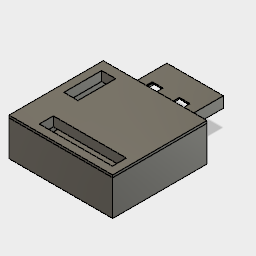
DigiCase (Autodesk Fusion 360 design; units mm, degrees)
Autodesk Fusion 360 part; units mm, degrees
sketch "Sketch1" plane through (0, 0, 0) normal (0, 1, 0) x (1, 0, 0)
  line L0 (0, 0) -> (-22, 0)
  line L1 (-22, 0) -> (-22, 20)
  line L2 (-22, 20) -> (-18, 20)
  line L3 (-18, 20) -> (-17, 20)
  line L4 (-5, 20) -> (0, 20)
  line L5 (0, 20) -> (0, 0)
  line L6 (-17, 20) -> (-5, 20)
  line L7 (-7.1, 21.5) -> (-7.1, 23.5)
  line L8 (-7.1, 23.5) -> (-9.35, 23.5)
  line L9 (-9.35, 23.5) -> (-9.35, 21.499)
  line L10 (-9.35, 21.499) -> (-7.1, 21.5)
  line L11 (-15.1, 21.5) -> (-15.1009, 23.4983)
  line L12 (-15.1009, 23.4983) -> (-12.8549, 23.4993)
  line L13 (-12.8549, 23.4993) -> (-12.854, 21.5032)
  line L14 (-12.854, 21.5032) -> (-15.1, 21.5)
  line L15 (-5.3006, 28.5) -> (-5.3006, 20)
  line L16 (-16.6958, 28.5) -> (-16.6958, 20)
  line L17 (-1.3, 19.5) -> (-1.3, 1.3)
  line L18 (-1.3, 1.3) -> (-20.7, 1.3)
  line L19 (-20.7, 1.3) -> (-20.7, 19.5)
  line L20 (-17.139, 1.5925) -> (-17.139, 4.5608)
  line L21 (-17.139, 4.5608) -> (-1.6625, 4.5608)
  line L22 (-1.6625, 4.5608) -> (-1.6625, 1.6)
  line L23 (-1.6625, 1.6) -> (-17.139, 1.5925)
  line L24 (-20.3439, 10.0007) -> (-20.3439, 18)
  line L25 (-20.3439, 18) -> (-17.3585, 18)
  line L26 (-17.3585, 18) -> (-17.3585, 10)
  line L27 (-17.3585, 10) -> (-20.3439, 10.0007)
  line L28 (-20.7, 19.5) -> (-1.3, 19.5)
  line L29 (-4.9026, 20) -> (-4.9026, 19.5)
  line L30 (-17.1025, 20) -> (-17.1025, 19.5)
  line L31 (-17, 20) -> (-17, 28.5)
  line L32 (-5, 20) -> (-5, 28.5)
  line L33 (-5, 28.5) -> (-17, 28.5)
  constraint perpendicular L0 L1
  constraint perpendicular L1 L2
  constraint perpendicular L1 L3
  constraint perpendicular L0 L5
  constraint coincident L6
  constraint perpendicular L6 L15
  constraint perpendicular L6 L16
  constraint perpendicular L17 L18
  constraint perpendicular L18 L19
  constraint vertical L20
  constraint perpendicular L20 L21
  constraint perpendicular L21 L22
  constraint perpendicular L24 L25
  constraint perpendicular L25 L26
  constraint coincident L4
  constraint coincident L3
  constraint coincident L28
  constraint perpendicular L28 L29
  constraint perpendicular L28 L30
  constraint perpendicular L6 L32
extrude "Extrude1" add sketch "Sketch1" along normal blind 0.5 contours L0 L1 L2 L3 L4 L5 L17 L18 L19 L28 L29 L30 | L3 L4 L6 L28 L29 L30 | L17 L18 L19 L28 makes body 1
extrude "Extrude2" add sketch "Sketch1" against normal blind 1.5 contours L17 L18 L19 L28 bodies 1
extrude "Extrude5" add sketch "Sketch1" along normal blind 1.5 separate body contours L0 L1 L2 L3 L4 L5 L17 L18 L19 L28 L29 L30 | L3 L4 L6 L28 L29 L30 | L17 L18 L19 L28 | L20 L21 L22 L23 | L24 L25 L26 L27 makes body 2
extrude "Extrude6" add sketch "Sketch1" along normal blind 7.5 contours L0 L1 L2 L3 L4 L5 L17 L18 L19 L28 L29 L30 bodies 2
move_body "MoveBody3" bodies 1 to x (1, 0, 0) y (0, 1, 0) z (0, 0, 1) at (0, 7.5, 0)
extrude "Extrude7" add sketch "Sketch1" along normal blind 4 separate body contours L3 L4 L6 L28 L29 L30 makes body 3
move_body "MoveBody4" bodies 3 to x (1, 0, 0) y (0, 1, 0) z (0, 0, 1) at (0, 3.5, 0)
combine "Combine1" operation add target body 3 tool bodies 1
extrude "Extrude8" add sketch "Sketch1" along normal blind 0.3 separate body contours L6 L15 L32 L33 | L6 L15 L16 L33 | L6 L16 L31 L33 makes body 4
move_body "MoveBody5" bodies 4 to x (1, 0, 0) y (0, 1, 0) z (0, 0, 1) at (0, 5.5, 0)
extrude "Extrude9" add sketch "Sketch1" along normal blind 2.3 separate body contours L6 L15 L32 L33 | L6 L16 L31 L33 makes body 5 at (-5.3006, 0.7667, -25.6667) makes body 6 at (-16.6958, 0.7667, -25.6667)
move_body "MoveBody6" bodies 5 6 to x (1, 0, 0) y (0, 1, 0) z (0, 0, 1) at (0, 3.5, 0)
combine "Combine2" operation add target body 5 tool bodies 4 6
combine "Combine3" operation add target body 3 tool bodies 5
